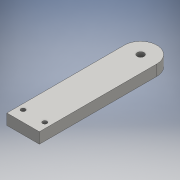
# Autodesk Inventor part: spool arm support
Saved by Autodesk Inventor 2016 SP1 (Build 200210100, 210)
## iProperties
Created: 2016-04-03
Part Number: spool arm support
Material: Generic
Document SubType Name: Modeling
Designer: ubik
Density: 1 g/cm^3
Appearance: Default
Author: ubik
Autodesk Inventor part; units mm, degrees
ref_plane "YZ Plane" through (0, 0, 0) normal (1, 0, 0) x (0, 1, 0)
ref_plane "XZ Plane" through (0, 0, 0) normal (0, 1, 0) x (-1, 0, 0)
ref_plane "XY Plane" through (0, 0, 0) normal (0, 0, 1) x (1, 0, 0)
sketch "Sketch1" plane through (0, 0, 0) normal (0, 0, 1) x (1, 0, 0)
  line L0 (14.9992, 46.0471) -> (14.9992, -62.4999)
  line L1 (14.9992, -62.4999) -> (-15, -62.5001)
  line L2 (-15, -62.5001) -> (-15, 46.2039)
  circle A0 centre (-0.0008, 46.0471) radius 3.2
  circle A1 centre (9.9992, -52.4999) radius 2
  circle A2 centre (-10, -52.5001) radius 2
  arc A3 (14.9992, 46.0471) -> (-15, 46.2039) centre (-0.0008, 46.0471) ccw
  point P0 (0, 0)
  point P1 (-4.1627, 60.4582)
  point P2 (4.1619, 60.4579)
  dimension "d2" = 62.5
  dimension "d3" = 15
  dimension "d4" = 6.4
  dimension "d5" = 15
  dimension "d7" = 4
  dimension "d8" = 4
  dimension "d9" = 5
  dimension "d10" = 10
  dimension "d11" = 10
  dimension "d12" = 5
  constraints: 6 end point, 4 centre point, 4 point on circle, 1 coincident, 1 parallel, 1 tangent
  measures "d2" distance from line of point (0, 0) L1
  measures "d3" distance from line of point (0, 0) L2
  measures "d4" diameter of A0
  measures "d5" distance from line of L0 A0.centre
  measures "d7" diameter of A1
  measures "d8" diameter of A2
  measures "d9" distance from line of L0 A1.centre
  measures "d10" distance from line of L1 A1.centre
  measures "d11" distance from line of L1 A2.centre
  measures "d12" distance from line of L2 A2.centre
extrude "Extrusion1" add sketch "Sketch1" along normal blind 10
equation "\"d2\" = 0.5 * d0"
equation "\"d3\" = 0.5 * d1"
equation "\"d5\" = 0.5 * d1"
equation "\"d11\" = d10"
equation "\"d12\" = d9"
equation "\"d1\" = 30"
equation "\"d0\" = 125"
body "Solid1"
